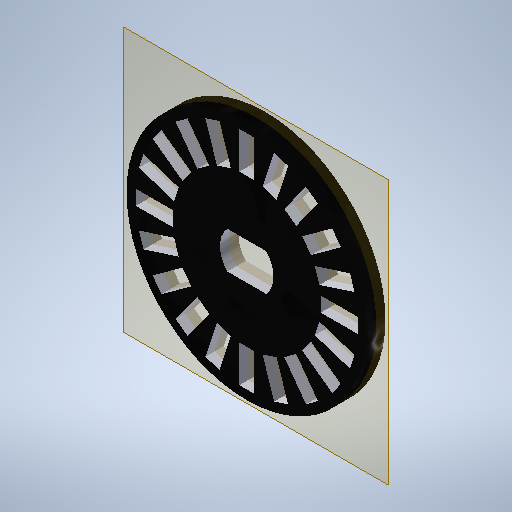
# Autodesk Inventor part: Encoder Disco-Novo-12-furos-04
Saved by Autodesk Inventor 2025 (Build 290162000, 162)
## iProperties
Created: 2016-09-28
Part Number: Encoder Disco-Novo-12-furos-04
Material: Genérico
Document SubType Name: Modeling
Designer: Marcelo Azevedo
Density: 1 g/cm^3
Appearance: Anodizado - Preto
Author: Marcelo Azevedo
Autodesk Inventor part; units mm, degrees
ref_plane "YZ Plane" through (0, 0, 0) normal (1, 0, 0) x (0, 1, 0)
ref_plane "XZ Plane" through (0, 0, 0) normal (0, 1, 0) x (-1, 0, 0)
ref_plane "XY Plane" through (0, 0, 0) normal (0, 0, 1) x (1, 0, 0)
sketch "Esboço1" plane through (0, 0, 0) normal (0, 1, 0) x (-1, 0, 0)
  line L0 (-2.1, 2) -> (2.1, 2)
  line L1 (-2.1, -2) -> (2.1, -2)
  arc A0 (-2.1, 2) -> (-2.1, -2) centre (0, 0) ccw
  arc A1 (2.1, -2) -> (2.1, 2) centre (0, 0) ccw
  circle A2 centre (0, 0) radius 13
  line L2 (0, -18.2) -> (0, 18.2) projected
  dimension "d2" = 2
  dimension "d3" = 2
  dimension "d4" = 2.9
  dimension "d5" = 2.9
  dimension "d40" = 2
  dimension "d41" = 26
  constraints: 4 end point, 4 point on circle, 3 centre point, 1 coincident, 1 horizontal, 1 midpoint, 1 parallel
  measures "d2" distance from line of A0.centre L1
  measures "d3" distance from line of point (0, 0) L0
  measures "d4" radius of A1
  measures "d5" radius of A0
  measures "d40" distance from line of L1 point (0, 0)
  measures "d41" diameter of A2
extrude "Extrusão4" add sketch "Esboço1" along normal blind 2 contours A0 L1 L2 A2 L0 | L2 A2 L1 A1 L0
sketch "Esboço17" plane through (0, 0, 0) normal (0, -1, 0) x (1, 0, 0)
  line L0 (-0.8, 12) -> (0.8, 12)
  line L1 (0.8, 12) -> (0.8, 8)
  line L2 (0.8, 8) -> (-0.8, 8)
  line L3 (-0.8, 8) -> (-0.8, 12)
  line L4 (0, 18.2) -> (0, -18.2) projected
  point P0 (0, 0)
  point P1 (0, 8)
  dimension "d114" = 8
  dimension "d115" = 4
  dimension "d116" = 0.8
  dimension "d117" = 0.8
  constraints: 8 end point, 2 parallel, 1 horizontal, 1 midpoint, 1 perpendicular
  measures "d114" distance of point (0, 8) point (0, 0)
  measures "d115" distance between parallel lines of L2 L0
  measures "d116" distance between parallel lines of L4 L1
  measures "d117" distance between parallel lines of L3 L4
extrude "Extrusão14" cut sketch "Esboço17" against normal through all
pattern_circular "Padrão circular10" count 20 over 360 about axis through (0, 0, 0) along (0, 1, 0) of "Extrusão14"
ref_plane "Plano de trabalho4" through (0, 1, 0) normal (0, -1, 0) x (1, 0, 0)
equation "\"d2\" = d40"
equation "\"d3\" = d40"
equation "\"d4\" = d5"
equation "\"d117\" = d116"
